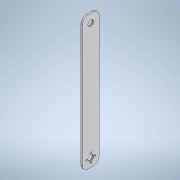
# Autodesk Inventor part: Arm Part
Saved by Autodesk Inventor 2020 (Build 240168000, 168)
## iProperties
Created: 2020-01-18
Part Number: Arm Part
Material: Generic
Document SubType Name: Modeling
Designer: kevin.nguyen
Density: 1 g/cm^3
Appearance: Default
Author: kevin.nguyen
Autodesk Inventor part; units mm, degrees
ref_plane "YZ Plane" through (0, 0, 0) normal (1, 0, 0) x (0, 1, 0)
ref_plane "XZ Plane" through (0, 0, 0) normal (0, 1, 0) x (-1, 0, 0)
ref_plane "XY Plane" through (0, 0, 0) normal (0, 0, 1) x (1, 0, 0)
sketch "Sketch1" plane through (0, 0, 0) normal (1, 0, 0) x (0, 1, 0)
  line L0 (0, 0) -> (0, -38.1)
  line L1 (0, -38.1) -> (304.8, -38.1)
  line L2 (304.8, -38.1) -> (304.8, 0)
  line L3 (304.8, 0) -> (0, 0)
  line L4 (0, 0) -> (38.1, 0) construction
  dimension "d0" = 38.1
  dimension "d1" = 90
  dimension "d2" = 304.8
  constraints: 10 end point, 2 parallel, 2 perpendicular, 1 horizontal, 1 vertical
  measures "d0" distance of L0.start L0.end
  measures "d1" angle of L0 L4
  measures "d2" distance of L1.end L0.end
extrude "Extrusion1" add sketch "Sketch1" along normal blind 3.2512
sketch "Sketch2" plane through (3.2512, 0, 0) normal (1, 0, 0) x (0, 0, -1)
  line L0 (0, 0) -> (38.1, 0) projected
  line L1 (19.05, 0) -> (19.05, 19.05)
  circle A0 centre (19.05, 19.05) radius 6.35
  line L2 (19.05, 19.05) -> (28.829, 19.05)
  line L3 (28.829, 19.05) -> (9.271, 19.05)
  circle A1 centre (9.271, 19.05) radius 1.778
  circle A2 centre (28.829, 19.05) radius 1.778
  line L4 (19.05, 19.05) -> (19.05, 28.829)
  line L5 (19.05, 28.829) -> (19.05, 9.271)
  circle A3 centre (19.05, 9.271) radius 1.778
  circle A4 centre (19.05, 28.829) radius 1.778
  line L6 (38.1, 304.8) -> (0, 304.8) projected
  line L7 (19.05, 304.8) -> (19.05, 285.75)
  circle A5 centre (19.05, 285.75) radius 6.35
  point P0 (38.1, 279.4)
  point P1 (0, 279.4)
  dimension "d5" = 19.05
  dimension "d6" = 12.7
  dimension "d7" = 9.779
  dimension "d8" = 19.558
  dimension "d9" = 3.556
  dimension "d10" = 3.556
  dimension "d11" = 9.779
  dimension "d12" = 19.558
  dimension "d13" = 3.556
  dimension "d14" = 3.556
  dimension "d17" = 19.05
  dimension "d18" = 12.7
  constraints: 12 end point, 6 centre point, 6 coincident, 2 point on line, 2 vertical, 1 horizontal, 1 midpoint, 1 perpendicular, 2 other
  measures "d5" distance of L1.start L1.end
  measures "d6" diameter of A0
  measures "d7" distance of L2.start L2.end
  measures "d8" distance of L2.end L3.end
  measures "d9" diameter of A1
  measures "d10" diameter of A2
  measures "d11" distance of L2.start L4.end
  measures "d12" distance of L4.end L5.end
  measures "d13" diameter of A3
  measures "d14" diameter of A4
  measures "d17" distance of L7.start L7.end
  measures "d18" diameter of A5
extrude "Extrusion2" cut sketch "Sketch2" against normal blind 25.4
fillet "Fillet1" radius 12.7 1 edges at (1.6256, 0, 0)
fillet "Fillet2" radius 12.7 2 edges at (1.6256, 304.8, 0) (1.6256, 304.8, -38.1)
fillet "Fillet3" radius 12.7 1 edges at (1.6256, 0, -38.1)
body "Solid1"
